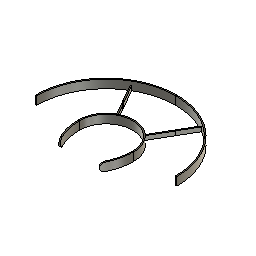
model (Autodesk Fusion 360 design; units mm, degrees)
Autodesk Fusion 360 part; units mm, degrees
sketch "Sketch1" plane through (0, 0, 0) normal (0, 0, 1) x (1, 0, 0)
  arc A0 (109.9852, 63.5) -> (-17.0148, 63.5) centre (46.4852, 63.5) ccw
  line L0 (-17.0148, 63.5) -> (109.9852, 63.5) construction
  arc A1 (-17.0148, 63.5) -> (0, 0) centre (109.9852, 63.5) ccw
  line L1 (46.4852, 63.5) -> (46.4852, 127) construction
  arc A2 (92.9705, 0) -> (109.9852, 63.5) centre (-17.0148, 63.5) ccw
  line L2 (46.4852, 63.5) -> (14.7352, 118.4926) construction
  arc A3 (95.5685, -1.5) -> (112.9852, 63.5) centre (-17.0148, 63.5) ccw
  arc A4 (112.9852, 63.5) -> (-20.0148, 63.5) centre (46.4852, 63.5) ccw
  arc A5 (-20.0148, 63.5) -> (-2.5981, -1.5) centre (109.9852, 63.5) ccw
  line L3 (-2.5981, -1.5) -> (0, 0)
  line L4 (92.9705, 0) -> (95.5685, -1.5)
  line L5 (14.7352, 118.4926) -> (-38.5015, 210.7014)
  line L6 (-38.5015, 210.7014) -> (-41.0996, 209.2014)
  line L7 (-41.0996, 209.2014) -> (12.1726, 116.9312)
  arc A6 (216.4852, 63.5) -> (-123.5148, 63.5) centre (46.4852, 63.5) ccw
  arc A7 (213.4852, 63.5) -> (-120.5148, 63.5) centre (46.4852, 63.5) ccw
  line L8 (-123.5148, 63.5) -> (-120.5148, 63.5)
  line L9 (213.4852, 63.5) -> (216.4852, 63.5)
  line L10 (-120.5148, 63.5) -> (-17.0148, 63.5) construction
  line L11 (109.9852, 63.5) -> (213.4852, 63.5) construction
  line L12 (134.0701, 209.2014) -> (80.7978, 116.9312)
  line L13 (78.2352, 118.4926) -> (131.472, 210.7014)
  line L14 (-14.4635, 163.0663) -> (-11.8832, 164.597) construction
  line L15 (-16.9635, 167.3964) -> (-15.6645, 168.1464)
  line L16 (-15.6645, 168.1464) -> (-10.6822, 159.5169)
  line L17 (-10.6822, 159.5169) -> (-9.3832, 160.2669)
  line L18 (-16.9635, 167.3964) -> (-13.1733, 163.8317) construction
  line L19 (-9.3832, 160.2669) -> (-13.1733, 163.8317) construction
  line L20 (109.934, 167.3964) -> (108.6349, 168.1464)
  line L21 (108.6349, 168.1464) -> (103.6526, 159.5169)
  line L22 (103.6526, 159.5169) -> (102.3536, 160.2669)
  line L23 (46.4852, 230.5) -> (46.4852, 233.5)
  dimension "d1" = 63.5
  dimension "d2" = 127
  dimension "d3" = 63.5
  dimension "d4" = 30
  dimension "d5" = 3
  dimension "d6" = 3
  dimension "d7" = 170
  dimension "d8" = -3
  dimension "d9" = 5
  constraint horizontal L0
  constraint midpoint A0.centre L0
  constraint tangent A0 A1
  constraint coincident A1.end L3.end
  constraint coincident A0.centre L1.start
  constraint midpoint A0 L1.end
  constraint symmetric A0.end L1 A0.start
  constraint symmetric A1.end L1 A2.start
  constraint symmetric A1 L1 A2
  constraint coincident A0 L2.end
  constraint parallel L2 L5
  constraint perpendicular L2 L6
  constraint coincident A0 L7.end
  constraint perpendicular L6 L7
  constraint horizontal L8
  constraint parallel L8 L9
  constraint coincident A0.end L0.start
  constraint parallel L0 L10
  constraint parallel L9 L11
  constraint coincident L6.end A6
  constraint symmetric L1 L2.end L13.start
  constraint symmetric L1 L5.end L13.end
  constraint symmetric L1 L6.end L12.start
  constraint symmetric L1 L7.end L12.end
  constraint midpoint L7 L14.start
  constraint midpoint L5 L14.end
  constraint coincident L7 L15.start
  constraint perpendicular L7 L15
  constraint perpendicular L15 L16
  constraint coincident L5 L17.end
  constraint perpendicular L5 L17
  constraint midpoint L14 L18.end
  constraint equal L18 L19
  constraint coincident L16 L18.end
  constraint symmetric L1 L15.start L20.start
  constraint symmetric L1 L15.end L20.end
  constraint symmetric L1 L16.end L21.end
  constraint symmetric L1 L17.end L22.end
  constraint midpoint A7 L23.start
  constraint midpoint A6 L23.end
  measures "d1" radius of A0
  measures "d2" radius of A1
  measures "d3" vertical distance of A0.end A1.end
  measures "d4" angle of L1 L2
  measures "d6" distance of L5 L7
  measures "d7" radius of A6
  measures "d9" distance of L14.start L15.start
extrude "Extrude1" add sketch "Sketch1" along normal blind 20 contours A0 A2 A3 A4 L4 L12 | A0 A4 L12 L13 | A0 A4 L5 L13 | A0 A4 L5 L7 | A0 A1 A4 A5 L3 L7 | L5 L6 L7 A7 | L5 L6 A6 A7 L23 | L7 A6 A7 L8 makes body 1 at (92.918, 111.1051, 13.3333) makes body 2 at (-122.745, 79.6595, 6.6667)
extrude "Extrude2" add sketch "Sketch1" along normal up to surface (20 mm away) separate body contours A6 A7 L9 L12 | A6 A7 L12 L23 makes body 3
extrude "Extrude3" add sketch "Sketch1" along normal blind 10 contours A7 L12 L13 L20 L21 L22 | L5 L7 A7 L15 L16 L17 bodies 2 3
extrude "Extrude4" add sketch "Sketch1" along normal up to surface (10 mm away) contours A4 L12 L13 L20 L21 L22 | A4 L5 L7 L15 L16 L17 bodies 1
fillet "Fillet1" radius 10 4 edges at (-1.299, -0.75, 20) (-1.299, -0.75, 0) (94.2695, -0.75, 20) (94.2695, -0.75, 0) on bodies 1
equation "d2 = d1 * 2"
equation "d3 = d1"
equation "d6 = d5"
